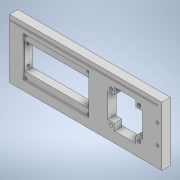
# Autodesk Inventor part: CubeBaseFront
Saved by Autodesk Inventor 2020 (Build 240168000, 168)
## iProperties
Created: 2019-12-01
Part Number: CubeBaseFront
Material: Generic
Document SubType Name: Modeling
Designer: torto
Density: 1 g/cm^3
Appearance: Default
Author: torto
Autodesk Inventor part; units mm, degrees
ref_plane "YZ Plane" through (0, 0, 0) normal (1, 0, 0) x (0, 1, 0)
ref_plane "XZ Plane" through (0, 0, 0) normal (0, 1, 0) x (-1, 0, 0)
ref_plane "XY Plane" through (0, 0, 0) normal (0, 0, 1) x (1, 0, 0)
sketch "Sketch1" plane through (0, 0, 0) normal (0, 0, 1) x (1, 0, 0)
  line L0 (0, 0) -> (228.6, 0)
  line L1 (228.6, 0) -> (228.6, 88.9)
  line L2 (228.6, 88.9) -> (0, 88.9)
  line L3 (0, 88.9) -> (0, 0)
  line L4 (228.6, 88.9) -> (222.25, 88.9) construction
  line L5 (222.25, 88.9) -> (222.25, 82.55) construction
  line L6 (222.25, 82.55) -> (228.6, 82.55) construction
  line L7 (228.6, 82.55) -> (228.6, 88.9) construction
  line L8 (222.25, 82.55) -> (0, 82.55)
  line L9 (0, 82.55) -> (0, 81.026)
  line L10 (0, 81.026) -> (222.25, 81.026)
  line L11 (222.25, 81.026) -> (222.25, 82.55)
  line L12 (228.6, 0) -> (222.25, 0) construction
  line L13 (222.25, 0) -> (222.25, 29.6333) construction
  line L14 (222.25, 29.6333) -> (228.6, 29.6333) construction
  line L15 (228.6, 29.6333) -> (228.6, 0) construction
  circle A0 centre (222.25, 29.6333) radius 2
  circle A1 centre (222.25, 59.2667) radius 2
  dimension "length" = 228.6
  dimension "height" = 88.9
  dimension "d3" = 6.35
  dimension "d4" = 6.35
  dimension "d5" = 222.25
  dimension "d6" = 1.524
  dimension "spacing" = 29.6333
  dimension "d9" = 6.35
  dimension "d10" = 4
  dimension "d13" = 29.6333
  constraints: 32 end point, 8 parallel, 4 horizontal, 4 perpendicular, 2 centre point, 2 coincident, 1 vertical, 3 other
  measures "length" distance of L2.end L1.end
  measures "height" distance of L1.end L0.end
  measures "d3" distance of L5.end L4.end
  measures "d4" distance of L5.end L6.end
  measures "d5" distance of L10.end L9.end
  measures "d6" distance of L9.end L8.end
  measures "spacing" distance of L12.end L13.end
  measures "d9" distance of L13.end L14.end
  measures "d10" diameter of A0
  measures "d13" distance of A0.centre A1.centre
extrude "Generic Shape" add sketch "Sketch1" along normal blind 12.7
sketch "Sketch2" plane through (0, 0, 12.7) normal (0, 0, 1) x (1, 0, 0)
  line L0 (228.6, 88.9) -> (0, 88.9) construction
  line L1 (228.6, 88.9) -> (222.25, 88.9) construction
  line L2 (222.25, 88.9) -> (222.25, 82.55) construction
  line L3 (222.25, 82.55) -> (228.6, 82.55) construction
  line L4 (228.6, 82.55) -> (228.6, 88.9) construction
  line L5 (222.25, 82.55) -> (0, 82.55)
  line L6 (0, 82.55) -> (0, 81.026)
  line L7 (0, 81.026) -> (222.25, 81.026)
  line L8 (222.25, 81.026) -> (222.25, 82.55)
  point P0 (0, 0)
  dimension "d21" = 6.35
  dimension "d22" = 6.35
  dimension "d23" = 222.25
  dimension "d24" = 1.524
  constraints: 16 end point, 4 parallel, 2 horizontal, 2 perpendicular
  measures "d21" distance of L2.end L1.end
  measures "d22" distance of L2.end L3.end
  measures "d23" distance of L7.end L6.end
  measures "d24" distance of L6.end L5.end
extrude "PCB Notch" cut sketch "Sketch2" against normal blind 6.35
sketch "Sketch4" plane through (0, 0, 0) normal (-1, 0, 0) x (0, 0, 1)
  line L0 (0, 0) -> (6.35, 0) construction
  line L1 (6.35, 0) -> (6.35, 29.6333) construction
  line L2 (6.35, 29.6333) -> (0, 29.6333) construction
  line L3 (0, 29.6333) -> (0, 0) construction
  circle A0 centre (6.35, 29.6333) radius 2
  line L4 (0, 88.9) -> (6.35, 88.9) construction
  line L5 (6.35, 88.9) -> (6.35, 59.2667) construction
  line L6 (6.35, 59.2667) -> (0, 59.2667) construction
  line L7 (0, 59.2667) -> (0, 88.9) construction
  circle A1 centre (6.35, 59.2667) radius 2
  dimension "d33" = 6.35
  dimension "d34" = 29.6333
  dimension "ScrewDiameter" = 4
  dimension "d36" = 6.35
  dimension "d37" = 29.6333
  dimension "d38" = 4
  constraints: 16 end point, 4 parallel, 2 centre point, 2 coincident, 2 horizontal, 2 perpendicular
  measures "d33" distance of L2.end L1.end
  measures "d34" distance of L1.end L0.end
  measures "ScrewDiameter" diameter of A0
  measures "d36" distance of L5.end L6.end
  measures "d37" distance of L4.end L5.end
  measures "d38" diameter of A1
extrude "2in Screw Depth" cut sketch "Sketch4" against normal blind 50.8
sketch "LCD" plane through (0, 0, 0) normal (0, 0, -1) x (-1, 0, 0)
  line L0 (0, 0) -> (-228.6, 0) construction
  line L1 (0, 0) -> (-69.85, 0) construction
  line L2 (-69.85, 0) -> (-69.85, 44.45) construction
  line L3 (-69.85, 44.45) -> (0, 44.45) construction
  line L4 (0, 44.45) -> (0, 0) construction
  line L5 (-118.4, 64.35) -> (-21.3, 64.35)
  line L6 (-21.3, 64.35) -> (-21.3, 24.55)
  line L7 (-21.3, 24.55) -> (-118.4, 24.55)
  line L8 (-118.4, 24.55) -> (-118.4, 64.35)
  line L9 (-118.4, 64.35) -> (-21.3, 24.55) construction
  line L10 (-21.3, 64.35) -> (-118.4, 24.55) construction
  line L11 (-118.975, 74.575) -> (-20.725, 74.575)
  line L12 (-20.725, 74.575) -> (-20.725, 14.325)
  line L13 (-20.725, 14.325) -> (-118.975, 14.325)
  line L14 (-118.975, 14.325) -> (-118.975, 74.575)
  line L15 (-118.975, 74.575) -> (-20.725, 14.325) construction
  line L16 (-20.725, 74.575) -> (-118.975, 14.325) construction
  dimension "d49" = 69.85
  dimension "d50" = 44.45
  dimension "LcdLength" = 97.1
  dimension "LcdHeight" = 39.8
  dimension "LcdBorderHeight" = 60.25
  dimension "LcdBorderLength" = 98.25
  constraints: 32 end point, 6 parallel, 4 midpoint, 3 horizontal, 3 perpendicular
  measures "d49" distance of L2.end L3.end
  measures "d50" distance of L1.end L2.end
  measures "LcdLength" distance of L6.end L7.end
  measures "LcdHeight" distance of L7.end L5.start
  measures "LcdBorderHeight" distance of L11.end L12.end
  measures "LcdBorderLength" distance of L12.end L13.end
extrude "LcdWindow" cut sketch "LCD" against normal blind 12.7 contours L5 L6 L7 L8
sketch "Sketch10" plane through (0, 0, 12.7) normal (0, 0, 1) x (1, 0, 0)
  line L0 (118.975, 74.575) -> (20.725, 74.575) projected
  line L1 (118.975, 14.325) -> (118.975, 74.575) projected
  line L2 (20.725, 14.325) -> (118.975, 14.325) projected
  line L3 (20.725, 74.575) -> (20.725, 14.325) projected
  point P0 (0, 0)
extrude "LcdFrame" cut sketch "Sketch10" against normal blind 1.64
sketch "LcdScrewsSketch" plane through (0, 0, 11.06) normal (0, 0, 1) x (1, 0, 0)
  line L0 (20.725, 14.325) -> (20.725, 74.575) construction
  line L1 (20.725, 74.575) -> (23.225, 74.575) construction
  line L2 (23.225, 74.575) -> (23.225, 72.075) construction
  line L3 (23.225, 72.075) -> (20.725, 72.075) construction
  line L4 (20.725, 72.075) -> (20.725, 74.575) construction
  circle A0 centre (23.225, 72.075) radius 1.5
  line L5 (20.725, 74.575) -> (118.975, 74.575) construction
  line L6 (69.85, 74.575) -> (69.85, 14.325) construction
  line L7 (118.975, 14.325) -> (20.725, 14.325) construction
  line L8 (20.725, 44.45) -> (118.975, 44.45) construction
  line L9 (118.975, 74.575) -> (118.975, 14.325) construction
  circle A1 centre (116.475, 72.075) radius 1.5
  circle A2 centre (23.225, 16.825) radius 1.5
  circle A3 centre (116.475, 16.825) radius 1.5
  point P0 (0, 0)
  dimension "LcdFrameHoleOffset" = 2.5
  dimension "d71" = 2.5
  dimension "LcdFrameHoleDiameter" = 3
  constraints: 12 end point, 4 centre point, 4 midpoint, 3 symmetric about line, 2 parallel, 1 coincident, 1 horizontal, 1 perpendicular, 3 other
  measures "LcdFrameHoleOffset" distance of L2.end L3.end
  measures "d71" distance of L1.end L2.end
  measures "LcdFrameHoleDiameter" diameter of A0
extrude "LcdScrews" cut sketch "LcdScrewsSketch" against normal blind 6
sketch "Sketch12" plane through (0, 0, 0) normal (0, 0, 1) x (1, 0, 0)
  line L0 (118.4, 24.55) -> (118.4, 64.35) construction
  line L1 (118.4, 44.45) -> (228.6, 44.45) construction
  line L2 (228.6, 0) -> (228.6, 88.9) construction
  line L3 (147.465, 72.9615) -> (199.535, 72.9615)
  line L4 (199.535, 72.9615) -> (199.535, 15.9385)
  line L5 (199.535, 15.9385) -> (147.465, 15.9385)
  line L6 (147.465, 15.9385) -> (147.465, 72.9615)
  line L7 (147.465, 72.9615) -> (199.535, 15.9385) construction
  line L8 (199.535, 72.9615) -> (147.465, 15.9385) construction
  point P0 (0, 0)
  point P1 (173.5, 44.45)
  dimension "InputHeight" = 57.023
  dimension "InputLength" = 52.07
  constraints: 14 end point, 5 midpoint, 2 parallel, 1 horizontal, 1 perpendicular
  measures "InputHeight" distance of L5.end L3.start
  measures "InputLength" distance of L4.end L5.end
extrude "InputCountersink" cut sketch "Sketch12" along normal blind 1.66
sketch "Sketch13" plane through (0, 0, 1.66) normal (0, 0, -1) x (-1, 0, 0)
  line L0 (-199.535, 15.9385) -> (-199.535, 72.9615) projected
  line L1 (-199.535, 72.9615) -> (-194.535, 72.9615) construction
  line L2 (-194.535, 72.9615) -> (-194.535, 67.9615) construction
  line L3 (-194.535, 67.9615) -> (-199.535, 67.9615) construction
  line L4 (-199.535, 67.9615) -> (-199.535, 72.9615) construction
  circle A0 centre (-194.535, 67.9615) radius 2.5
  line L5 (-199.535, 72.9615) -> (-147.465, 72.9615) projected
  line L6 (-173.5, 72.9615) -> (-173.5, 15.9385) construction
  line L7 (-147.465, 15.9385) -> (-199.535, 15.9385) projected
  line L8 (-199.535, 44.45) -> (-147.465, 44.45) construction
  line L9 (-147.465, 72.9615) -> (-147.465, 15.9385) projected
  line L10 (-199.535, 72.9615) -> (-189.535, 72.9615) construction
  line L11 (-189.535, 72.9615) -> (-189.535, 62.9615)
  line L12 (-189.535, 62.9615) -> (-199.535, 62.9615)
  line L13 (-199.535, 62.9615) -> (-199.535, 72.9615) construction
  circle A1 centre (-152.465, 67.9615) radius 2.5
  line L14 (-157.465, 72.9615) -> (-157.465, 62.9615)
  line L15 (-157.465, 62.9615) -> (-147.465, 62.9615)
  circle A2 centre (-194.535, 20.9385) radius 2.5
  line L16 (-189.535, 15.9385) -> (-189.535, 25.9385)
  line L17 (-189.535, 25.9385) -> (-199.535, 25.9385)
  circle A3 centre (-152.465, 20.9385) radius 2.5
  line L18 (-157.465, 25.9385) -> (-147.465, 25.9385)
  line L19 (-157.465, 15.9385) -> (-157.465, 25.9385)
  point P0 (0, 0)
  dimension "InputHoleSpacing" = 5
  dimension "d80" = 5
  dimension "InputScrewDiameter" = 5
  dimension "d82" = 10
  dimension "d83" = 10
  constraints: 32 end point, 12 symmetric about line, 4 centre point, 4 midpoint, 4 parallel, 2 horizontal, 2 perpendicular, 1 coincident, 3 other
  measures "InputHoleSpacing" distance of L2.end L3.end
  measures "d80" distance of L1.end L2.end
  measures "InputScrewDiameter" diameter of A0
  measures "d82" distance of L11.end L12.end
  measures "d83" distance of L10.end L11.end
extrude "InputCut" cut sketch "Sketch13" against normal blind 11.04 contours L0 L12 L11 L5 L14 L15 L9 L18 L19 L7 L16 L17
extrude "Extrusion11" cut sketch "Sketch13" against normal blind 11.04 contours A0 | A1 | A2 | A3
equation "\"d3\" = 0.5 * thickness"
equation "\"d4\" = 0.5 * thickness"
equation "\"d5\" = length - 0.5 * thickness"
equation "\"spacing\" = 0.333333 * height"
equation "\"d9\" = 0.5 * thickness"
equation "\"d10\" = ScrewDiameter"
equation "\"d13\" = spacing"
equation "\"d25\" = 0.5 * thickness"
equation "\"d33\" = 0.5 * thickness"
equation "\"d34\" = 0.333333 * height"
equation "\"d36\" = 0.5 * thickness"
equation "\"d37\" = 0.333333 * height"
equation "\"d38\" = ScrewDiameter"
equation "\"d49\" = 0.333333 * length - 0.5 * thickness"
equation "\"d50\" = 0.5 * height"
equation "\"d66\" = thickness"
equation "\"d71\" = LcdFrameHoleOffset"
equation "\"d80\" = InputHoleSpacing"
equation "\"d82\" = 2 * InputHoleSpacing"
equation "\"d83\" = 2 * InputHoleSpacing"
equation "\"d84\" = thickness - InputThickness"
equation "\"d86\" = thickness - InputThickness"
equation "\"thickness\" = 12.7"
equation "\"InputThickness\" = 1.66"
body "Solid1"
